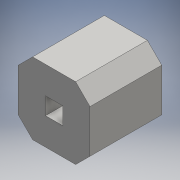
# Autodesk Inventor part: Pin Shroud
Saved by Autodesk Inventor 2016 (Build 200138000, 138)
## iProperties
Created: 2016-04-16
Part Number: Pin Shroud
Material: Generic
Document SubType Name: Modeling
Designer: Jarrett
Density: 1 g/cm^3
Appearance: Default
Author: Jarrett
Autodesk Inventor part; units mm, degrees
ref_plane "YZ Plane" through (0, 0, 0) normal (1, 0, 0) x (0, 1, 0)
ref_plane "XZ Plane" through (0, 0, 0) normal (0, 1, 0) x (-1, 0, 0)
ref_plane "XY Plane" through (0, 0, 0) normal (0, 0, 1) x (1, 0, 0)
sketch "Sketch1" plane through (0, 0, 0) normal (0, 1, 0) x (-1, 0, 0)
  line L0 (0, 0) -> (2.5, 0)
  line L1 (2.5, 0) -> (2.5, -2.5)
  line L2 (2.5, -2.5) -> (0, -2.5)
  line L3 (0, -2.5) -> (0, 0)
  dimension "d0" = 2.5
  constraints: 8 end point, 2 parallel, 2 perpendicular, 1 horizontal
  measures "d0" distance of L0.end L1.end
extrude "Extrusion1" add sketch "Sketch1" along normal blind 2.5
chamfer "Chamfer1" distance 0.5 angle 45 4 edges at (0, 1.25, 0) (-2.5, 1.25, 0) (0, 1.25, -2.5) (-2.5, 1.25, -2.5)
sketch "Sketch2" plane through (0, 2.5, 0) normal (0, 1, 0) x (1, 0, 0)
  line L0 (-0.5, 0) -> (-2, 0) projected
  line L1 (-1.25, 0) -> (-1.25, 2.5) construction
  line L2 (-2, 2.5) -> (-0.5, 2.5) projected
  line L3 (-2.5, 0.5) -> (-2.5, 2) projected
  line L4 (-2.5, 1.25) -> (0, 1.25) construction
  line L5 (0, 0.5) -> (0, 2) projected
  line L6 (-0.95, 0.95) -> (-1.55, 0.95)
  line L7 (-1.55, 0.95) -> (-1.55, 1.55)
  line L8 (-1.55, 1.55) -> (-0.95, 1.55)
  line L9 (-0.95, 1.55) -> (-0.95, 0.95)
  line L10 (-0.95, 0.95) -> (-1.55, 1.55) construction
  line L11 (-1.55, 0.95) -> (-0.95, 1.55) construction
  point P0 (0, 0)
  point P1 (-1.25, 1.25)
  dimension "d6" = 0.6
  constraints: 16 end point, 7 midpoint, 2 parallel, 2 perpendicular, 1 horizontal
  measures "d6" distance of L6.end L7.end
extrude "Extrusion2" cut sketch "Sketch2" against normal up to next
body "Solid1"
